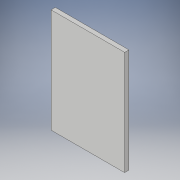
# Autodesk Inventor part: HX711 Mount Lid v1.2
Saved by Autodesk Inventor 2019 (Build 230136000, 136)
## iProperties
Created: 2020-01-31
Part Number: HX711 Mount Lid v1.2
Material: Generic
Document SubType Name: Modeling
Designer: Obscure_Decision
Density: 1 g/cm^3
Appearance: Default
Author: Obscure_Decision
Autodesk Inventor part; units mm, degrees
ref_plane "YZ Plane" through (0, 0, 0) normal (1, 0, 0) x (0, 1, 0)
ref_plane "XZ Plane" through (0, 0, 0) normal (0, 1, 0) x (-1, 0, 0)
ref_plane "XY Plane" through (0, 0, 0) normal (0, 0, 1) x (1, 0, 0)
sketch "Sketch1" plane through (0, 0, 0) normal (0, 0, 1) x (1, 0, 0)
  line L0 (-14.2005, -20.11) -> (14.2005, -20.11)
  line L1 (14.2005, -20.11) -> (14.2005, 20.11)
  line L2 (14.2005, 20.11) -> (-14.2005, 20.11)
  line L3 (-14.2005, 20.11) -> (-14.2005, -20.11)
  line L4 (-14.2005, -20.11) -> (14.2005, 20.11) construction
  line L5 (14.2005, -20.11) -> (-14.2005, 20.11) construction
  point P0 (0, 0)
  dimension "d0" = 40.22
  dimension "d1" = 28.401
  constraints: 12 end point, 2 midpoint, 2 parallel, 1 horizontal, 1 perpendicular
  measures "d0" distance of L1.end L0.end
  measures "d1" distance of L1.end L2.end
extrude "Extrusion1" add sketch "Sketch1" along normal blind 1.656
body "Solid1"
